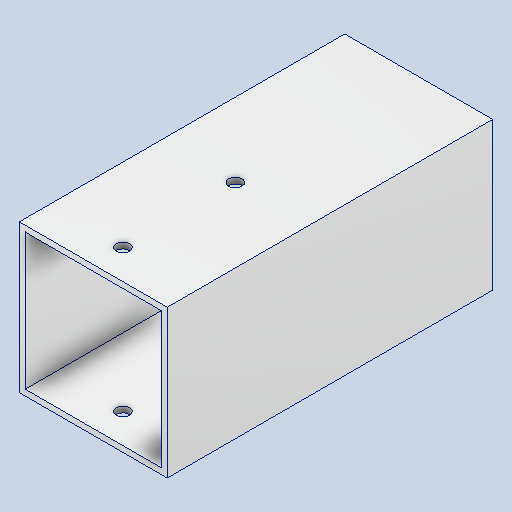
# Autodesk Inventor part: center
Saved by Autodesk Inventor 2022 (Build 260153000, 153)
## iProperties
Created: 2022-10-09
Part Number: center
Material: アルミニウム 6061
Document SubType Name: Modeling
Designer: haya
Density: 2.7 g/cm^3
Appearance: アルミニウム - フラット
Mass: 113.704 g
Surface Area: 429.939 cm^2
Volume: 42.1128 cm^3
Author: haya
Autodesk Inventor part; units mm, degrees
ref_plane "YZ Plane" through (0, 0, 0) normal (1, 0, 0) x (0, 1, 0)
ref_plane "XZ Plane" through (0, 0, 0) normal (0, 1, 0) x (-1, 0, 0)
ref_plane "XY Plane" through (0, 0, 0) normal (0, 0, 1) x (1, 0, 0)
sketch "スケッチ1" plane through (0, 0, 0) normal (0, 0, 1) x (1, 0, 0)
  line L0 (0, 0) -> (50, 0)
  line L1 (50, 0) -> (50, 50)
  line L2 (50, 50) -> (0, 50)
  line L3 (0, 50) -> (0, 0)
  line L4 (2, 48) -> (48, 48)
  line L5 (48, 48) -> (48, 2)
  line L6 (48, 2) -> (2, 2)
  line L7 (2, 2) -> (2, 48)
  dimension "d0" = 50
  dimension "d1" = 50
  dimension "d2" = 2
  constraints: 16 end point, 4 parallel, 2 perpendicular, 1 horizontal, 3 other
  measures "d0" distance of L2.end L0.start
  measures "d1" distance of L0.start L0.end
  measures "d2" distance between parallel lines of L0 L6
extrude "押し出し1" add sketch "スケッチ1" along normal blind 110
sketch "スケッチ5" plane through (0, 50, 0) normal (0, 1, 0) x (1, 0, 0)
  line L0 (50, 0) -> (0, 0) projected
  line L1 (0, 0) -> (0, -110) projected
  line L2 (50, -110) -> (0, -110) projected
  line L3 (50, 0) -> (50, -110) projected
  line L4 (25, 0) -> (25, -110) construction
  point P0 (0, 0)
  point P1 (25, -62)
  point P2 (25, -100)
  dimension "d42" = 38
  dimension "d43" = 10
  constraints: 2 end point, 2 midpoint, 2 point on line
  measures "d42" distance of point (25, -100) point (25, -62)
  measures "d43" distance from line of point (25, -100) L2
hole "穴4" at (25, 50, 62) at (25, 50, 100) direction (0, -1, 0) diameter 4.5 end through all
